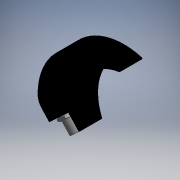
# Autodesk Inventor part: SCHUNK-Stecker 2 ERD
Saved by Autodesk Inventor 2017.3 (Build 213256000, 256)
## iProperties
Part Number: SCHUNK-Stecker 2 ERD
Material: Generic
Catalog Web Link: www.cadenas.de
Description: Stecker 2-Miniature rotary unit
Vendor: SCHUNK
Document SubType Name: Modeling
Designer: partserver
Manufacturer: SCHUNK
Mass: 9.01845 g
Surface Area: 45.5668 cm^2
Volume: 9.01845 cm^3
Density: 1 g/cm^3
Appearance: PSOLRGB-0-0-0
Category: PARTsolutions
Company: SCHUNK
Title: SCHUNK-Stecker 2 ERD
Author: Cadenas PARTsolutions
Comments: Miniature rotary unit
PSOL_IDENT_0: {$CADENAS_DATA\23d-libs\schunk\greifsysteme\drehmodule\drehmodule_elektrisch\schwenkeinheiten\miniat
PSOL_IDENT_1: ur_schwenkeinheiten\erd_stk_2.prj},183 {VTYP=3D},{NB=SCHUNK-Stecker 2 ERD},{LINA=SCHUNK-Stecker 2 ER
PSOL_IDENT_2: D},{NN=Stecker 2},{DATE=23.04.2020 15:23:31},{GEOMDATE=04.12.2019 08:06:04},{VERSION=},{LINEID=10},{
PSOL_IDENT_3: WBVAR=},{WBNUMERIC=}  {NB=SCHUNK-Stecker 2 ERD},{LINA=SCHUNK-Stecker 2 ERD},{KT=DUMMY},{TYP=ERD},{KH=
PSOL_IDENT_4: 44.500},{KB=12.000},{KD1=55.000},{KD2=69.000},{KP1=13.500},{KP2=5.000},{KP3=40.800},{KP4=14.000},{KP
PSOL_IDENT_5: 5=34.300},{KW=43.000},{KR=8.000},{BD1=6.000},{BT1=23.000},{BT2=35.000},{BA1=28.000},{BA2=19.500},{SD
PSOL_IDENT_6: 1=5.500},{SD2=2.500},{ST1=3.000},{ST2=1.300},{SBP1=1.700},{SBP2=1.700},{SBP3=0.200},{SBP4=1.200},{SB
PSOL_IDENT_7: P5=1.800},{SBP6=0.700},{SBP7=1.300},{SBP8=0.400},{SBD=1.000},{STD1=8.700},{STD2=8.000},{STD3=6.000},
PSOL_IDENT_8: {STD4=11.500},{STT1=9.200},{STT2=8.500},{STT3=7.500},{STT4=6.500},{STT5=0.800},{SW=10.000},{BT3=15.5
PSOL_IDENT_9: 00},{BD2=8.200},{BA3=4.500}
NB: SCHUNK-Stecker 2 ERD
NN: Stecker 2
NT: Miniature rotary unit
NBSYN: SCHUNK-Stecker 2 $TYP.
LINA: SCHUNK-Stecker 2 ERD
CATALOG: SCHUNK
TYP: ERD
KH: 44.5
KB: 12
KD1: 55
KD2: 69
KP1: 13.5
KP2: 5
KP3: 40.8
KP4: 14
KP5: 34.3
KW: 43
KR: 8
BD1: 6
BT1: 23
BT2: 35
BA1: 28
BA2: 19.5
SD1: 5.5
SD2: 2.5
ST1: 3
ST2: 1.3
SBP1: 1.7
SBP2: 1.7
SBP3: 0.2
SBP4: 1.2
SBP5: 1.8
SBP6: 0.7
SBP7: 1.3
SBP8: 0.4
SBD: 1
STD1: 8.7
STD2: 8
STD3: 6
STD4: 11.5
STT1: 9.2
STT2: 8.5
STT3: 7.5
STT4: 6.5
STT5: 0.8
SW: 10
BT3: 15.5
BD2: 8.2
BA3: 4.5
SUPPLIER: SCHUNK
ARTICLENO: SCHUNK-Stecker 2 ERD
BOMINFO: SCHUNK-Stecker 2 ERD
CREATOR: CADENAS GmbH
Autodesk Inventor part; units mm, degrees
sketch "Sketch_1" plane through (0, 0, 0) normal (0, 1, 0) x (-1, 0, 0)
  arc A0 (-4.0163, -28.1709) -> (-4.0796, -27.1957) centre (-4.1538, -27.6902) ccw
  arc A1 (-25.3266, 10.715) -> (-4.0796, -27.1957) centre (0, 0) ccw
  arc A2 (-25.3266, 10.715) -> (-26.1528, 11.2508) centre (-25.7871, 10.9098) ccw
  line L0 (-26.1528, 11.2508) -> (-31.5603, 5.452)
  line L1 (-31.5603, 5.452) -> (-41.7992, 15)
  line L2 (-41.7992, 15) -> (-45.8501, 10.656)
  arc A3 (-45.8501, 10.656) -> (-47.999, 5.2604) centre (-39.9992, 5.2) ccw
  arc A4 (-47.999, 5.2604) -> (-4.0163, -28.1709) centre (-13.5, 5) ccw
  constraints: 10 point on circle, 6 end point, 5 centre point
extrude "Extrusion1" add sketch "Sketch_1" along normal blind 12
sketch "Sketch_2" plane through (0, 6, 0) normal (0, 1, 0) x (1, 0, 0)
  line L0 (40, 23) -> (23.9489, 23)
  line L1 (23.9489, 23) -> (24.7, 24.25)
  line L2 (24.7, 24.25) -> (25.8, 24.25)
  line L3 (25.8, 24.25) -> (26, 24.45)
  line L4 (26, 24.45) -> (26, 25.45)
  arc A0 (26, 25.45) -> (25.7, 25.75) centre (25.7, 25.45) ccw
  line L5 (25.7, 25.75) -> (23, 25.75)
  line L6 (23, 25.75) -> (23, 26)
  line L7 (23, 26) -> (40, 26)
  line L8 (40, 26) -> (40, 23)
  line L9 (40, 23) -> (23.9489, 23)
  constraints: 20 end point, 2 point on circle, 1 centre point
revolve "Revolution1" cut sketch "Sketch_2" angle 360 about axis through (40, 6, -23) along (1, 0, 0)
sketch "Sketch_3" plane through (0, 6, 0) normal (0, 1, 0) x (1, 0, 0)
  line L0 (45, 14.5) -> (35.9489, 14.5)
  line L1 (35.9489, 14.5) -> (36.7, 15.75)
  line L2 (36.7, 15.75) -> (37.8, 15.75)
  line L3 (37.8, 15.75) -> (38, 15.95)
  line L4 (38, 15.95) -> (38, 16.95)
  arc A0 (38, 16.95) -> (37.7, 17.25) centre (37.7, 16.95) ccw
  line L5 (37.7, 17.25) -> (35, 17.25)
  line L6 (35, 17.25) -> (35, 17.5)
  line L7 (35, 17.5) -> (45, 17.5)
  line L8 (45, 17.5) -> (45, 14.5)
  line L9 (45, 14.5) -> (35.9489, 14.5)
  constraints: 20 end point, 2 point on circle, 1 centre point
revolve "Revolution2" cut sketch "Sketch_3" angle 360 about axis through (45, 6, -14.5) along (1, 0, 0)
sketch "Sketch_4" plane through (26, 6, -23) normal (1, 0, 0) x (0, 0, -1)
  line L0 (-1.25, -0.7217) -> (0, -1.4434)
  line L1 (0, -1.4434) -> (1.25, -0.7217)
  line L2 (1.25, -0.7217) -> (1.25, 0.7217)
  line L3 (1.25, 0.7217) -> (0, 1.4434)
  line L4 (0, 1.4434) -> (-1.25, 0.7217)
  line L5 (-1.25, 0.7217) -> (-1.25, -0.7217)
  constraints: 12 end point
sketch "Sketch_5" plane through (38, 6, -14.5) normal (1, 0, 0) x (0, 0, -1)
  line L0 (-1.25, -0.7217) -> (0, -1.4434)
  line L1 (0, -1.4434) -> (1.25, -0.7217)
  line L2 (1.25, -0.7217) -> (1.25, 0.7217)
  line L3 (1.25, 0.7217) -> (0, 1.4434)
  line L4 (0, 1.4434) -> (-1.25, 0.7217)
  line L5 (-1.25, 0.7217) -> (-1.25, -0.7217)
  constraints: 12 end point
extrude "Extrusion2" cut sketch "Sketch_4" against normal blind 1.3
extrude "Extrusion3" cut sketch "Sketch_5" against normal blind 1.3
sketch "Sketch_6" plane through (0, 6, 0) normal (0, 1, 0) x (1, 0, 0)
  line L0 (31.794, -16.1984) -> (37.0454, -10.567)
  line L1 (37.0454, -10.567) -> (40.5194, -13.8065)
  line L2 (40.5194, -13.8065) -> (40.857, -14.9107)
  line L3 (40.857, -14.9107) -> (40.2805, -15.529)
  line L4 (40.2805, -15.529) -> (39.1554, -15.2692)
  line L5 (39.1554, -15.2692) -> (38.8628, -14.9964)
  line L6 (38.8628, -14.9964) -> (34.6411, -19.5237)
  line L7 (34.6411, -19.5237) -> (34.2033, -19.539)
  line L8 (34.2033, -19.539) -> (34.1739, -19.5115)
  line L9 (34.1739, -19.5115) -> (39.2889, -14.0264)
  line L10 (39.2889, -14.0264) -> (38.5575, -13.3444)
  line L11 (38.5575, -13.3444) -> (33.9881, -18.2444)
  line L12 (33.9881, -18.2444) -> (31.794, -16.1984)
  line L13 (31.794, -16.1984) -> (37.0454, -10.567)
  constraints: 28 end point
revolve "Revolution3" add sketch "Sketch_6" angle 360 about axis through (31.794, 6, 16.1984) along (-0.6819984, 0, 0.7313537)
sketch "Sketch7" plane through (31.794, 6, 16.1984) normal (-0.6819984, 0, 0.7313537) x (0.7313537, 0, 0.6819984)
  point P0 (1.8, 0.2)
hole "Hole1" at (33.1105, 6.2, 17.426) direction (0.6819984, 0, -0.7313537) diameter 1 depth 9.2
sketch "Flanschdosenbohrungen_Sketch_7_0" plane through (-2.2922, 4.8, -2.0874) normal (0, 1, 0) x (1, 0, 0)
  line L0 (33.1105, -17.426) -> (39.3849, -10.6976)
  line L1 (39.3849, -10.6976) -> (39.7505, -11.0386)
  line L2 (39.7505, -11.0386) -> (33.4762, -17.767)
  line L3 (33.4762, -17.767) -> (33.1105, -17.426)
  line L4 (33.1105, -17.426) -> (39.3849, -10.6976)
  constraints: 10 end point
revolve "Revolution4" cut sketch "Flanschdosenbohrungen_Sketch_7_0" angle 360 about axis through (30.8183, 4.8, 15.3387) along (-0.6819984, 0, 0.7313537)
sketch "Flanschdosenbohrungen_Sketch_7_1" plane through (-0.8295, 4.3, -0.7234) normal (0, 1, 0) x (1, 0, 0)
  line L0 (33.1105, -17.426) -> (39.3849, -10.6976)
  line L1 (39.3849, -10.6976) -> (39.7505, -11.0386)
  line L2 (39.7505, -11.0386) -> (33.4762, -17.767)
  line L3 (33.4762, -17.767) -> (33.1105, -17.426)
  line L4 (33.1105, -17.426) -> (39.3849, -10.6976)
  constraints: 10 end point
revolve "Revolution5" cut sketch "Flanschdosenbohrungen_Sketch_7_1" angle 360 about axis through (32.281, 4.3, 16.7027) along (-0.6819984, 0, 0.7313537)
sketch "Flanschdosenbohrungen_Sketch_7_2" plane through (-1.0489, 7.7, -0.928) normal (0, 1, 0) x (1, 0, 0)
  line L0 (33.1105, -17.426) -> (39.3849, -10.6976)
  line L1 (39.3849, -10.6976) -> (39.7505, -11.0386)
  line L2 (39.7505, -11.0386) -> (33.4762, -17.767)
  line L3 (33.4762, -17.767) -> (33.1105, -17.426)
  line L4 (33.1105, -17.426) -> (39.3849, -10.6976)
  constraints: 10 end point
revolve "Revolution6" cut sketch "Flanschdosenbohrungen_Sketch_7_2" angle 360 about axis through (32.0616, 7.7, 16.4981) along (-0.6819984, 0, 0.7313537)
sketch "Sketch_9" plane through (6.6836, 0, -7.1673) normal (0.6819984, 0, -0.7313537) x (-0.7313537, 0, -0.6819984)
  circle A0 centre (-34.3, 6) radius 6
  line L0 (-40.0735, 6) -> (-37.1868, 1)
  line L1 (-37.1868, 1) -> (-31.4132, 1)
  line L2 (-31.4132, 1) -> (-28.5265, 6)
  line L3 (-28.5265, 6) -> (-31.4132, 11)
  line L4 (-31.4132, 11) -> (-37.1868, 11)
  line L5 (-37.1868, 11) -> (-40.0735, 6)
  constraints: 12 end point, 1 centre point
extrude "Extrusion4" cut sketch "Sketch_9" along normal blind 7.6
sketch "Sketch_10" plane through (0, 6, 0) normal (0, 1, 0) x (1, 0, 0)
  line L0 (51.1453, 11.1515) -> (42.1417, 1.4964)
  line L1 (42.1417, 1.4964) -> (41.4986, 3.7393)
  line L2 (41.4986, 3.7393) -> (42.5216, 4.8363)
  line L3 (42.5216, 4.8363) -> (42.4969, 5.543)
  line L4 (42.4969, 5.543) -> (41.6924, 6.2932)
  line L5 (41.6924, 6.2932) -> (40.9858, 6.2685)
  line L6 (40.9858, 6.2685) -> (48.1468, 13.9477)
  line L7 (48.1468, 13.9477) -> (51.1453, 11.1515)
  line L8 (51.1453, 11.1515) -> (42.1417, 1.4964)
  constraints: 18 end point
revolve "Revolution7" cut sketch "Sketch_10" angle 360 about axis through (51.1453, 6, -11.1515) along (0.6819984, 0, -0.7313537)
sketch "Sketch_11" plane through (44.3253, 6, -3.838) normal (0.6819984, 0, -0.7313537) x (-0.7313537, 0, -0.6819984)
  line L0 (-2, -1.1547) -> (0, -2.3094)
  line L1 (0, -2.3094) -> (2, -1.1547)
  line L2 (2, -1.1547) -> (2, 1.1547)
  line L3 (2, 1.1547) -> (0, 2.3094)
  line L4 (0, 2.3094) -> (-2, 1.1547)
  line L5 (-2, 1.1547) -> (-2, -1.1547)
  constraints: 12 end point
extrude "Extrusion5" cut sketch "Sketch_11" against normal blind 2
ref_plane "welle_XY" through (0, 6, 0) normal (0, 1, 0) x (1, 0, 0)
ref_plane "welle_YZ" through (0, 6, 0) normal (1, 0, 0) x (0, 0, -1)
ref_plane "welle_ZX" through (0, 6, 0) normal (0, 0, -1) x (0, 1, 0)
body "Solid1"
